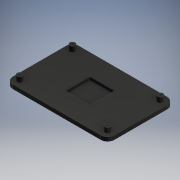
# Autodesk Inventor part: BackBracket
Saved by Autodesk Inventor 2018 (Build 220112000, 112)
## iProperties
Created: 2020-01-28
Part Number: BackBracket
Material: Steel, Mild
Document SubType Name: Modeling
Designer: Bradley
Density: 7.85 g/cm^3
Appearance: Glossy - Black
Author: Bradley
Autodesk Inventor part; units mm, degrees
ref_plane "YZ Plane" through (0, 0, 0) normal (1, 0, 0) x (0, 1, 0)
ref_plane "XZ Plane" through (0, 0, 0) normal (0, 1, 0) x (-1, 0, 0)
ref_plane "XY Plane" through (0, 0, 0) normal (0, 0, 1) x (1, 0, 0)
sketch "Sketch1" plane through (0, 0, 0) normal (0, 0, 1) x (1, 0, 0)
  line L0 (-45, -34) -> (45, -34)
  line L1 (52, -27) -> (52, 27)
  line L2 (45, 34) -> (-45, 34)
  line L3 (-52, 27) -> (-52, -27)
  line L4 (-52, -34) -> (52, 34) construction
  line L5 (52, -34) -> (-52, 34) construction
  line L6 (-45, 27) -> (45, 27) construction
  line L7 (45, 27) -> (45, -27) construction
  line L8 (45, -27) -> (-45, -27) construction
  line L9 (-45, -27) -> (-45, 27) construction
  arc A0 (-45, 34) -> (-52, 27) centre (-45, 27) ccw
  arc A1 (52, 27) -> (45, 34) centre (45, 27) ccw
  arc A2 (45, -34) -> (52, -27) centre (45, -27) ccw
  arc A3 (-52, -27) -> (-45, -34) centre (-45, -27) ccw
  point P0 (0, 0)
  dimension "d0" = 104
  dimension "d1" = 68
  dimension "d2" = 54
  dimension "d3" = 90
  constraints: 20 end point, 8 point on circle, 8 point on line, 8 tangent, 4 centre point, 4 parallel, 3 equal radius, 2 midpoint, 2 perpendicular, 1 coincident, 1 horizontal, 3 other
  measures "d0" distance of L5.end L4.end
  measures "d1" distance of L4.end L5.start
  measures "d2" distance of L8.end L6.start
  measures "d3" distance of L6.start L6.end
extrude "Extrusion1" add sketch "Sketch1" along normal mid plane 4
sketch "Sketch2" plane through (0, 0, 2) normal (0, 0, 1) x (1, 0, 0)
  line L0 (45, 34) -> (-45, 34) projected
  arc A0 (-45, 34) -> (-52, 27) centre (-45, 27) ccw projected
  line L1 (-52, 27) -> (-52, -27) projected
  arc A1 (-52, -27) -> (-45, -34) centre (-45, -27) ccw projected
  line L2 (-45, -34) -> (45, -34) projected
  arc A2 (45, -34) -> (52, -27) centre (45, -27) ccw projected
  line L3 (52, -27) -> (52, 27) projected
  arc A3 (52, 27) -> (45, 34) centre (45, 27) ccw projected
  circle A4 centre (-45, 27) radius 2.75
  circle A5 centre (45, 27) radius 2.75
  circle A6 centre (45, -27) radius 2.75
  circle A7 centre (-45, -27) radius 2.75
  point P0 (0, 0)
  dimension "d7" = 5.5
  constraints: 4 centre point, 4 coincident, 3 equal radius
  measures "d7" diameter of A4
extrude "Extrusion2" add sketch "Sketch2" along normal blind 5.3 contours A4 | A5 | A6 | A7
sketch "Sketch3" plane through (0, 0, -2) normal (0, 0, -1) x (-1, 0, 0)
  line L0 (45, 34) -> (-45, 34) projected
  arc A0 (-45, 34) -> (-52, 27) centre (-45, 27) ccw projected
  line L1 (-52, 27) -> (-52, -27) projected
  arc A1 (-52, -27) -> (-45, -34) centre (-45, -27) ccw projected
  line L2 (-45, -34) -> (45, -34) projected
  arc A2 (45, -34) -> (52, -27) centre (45, -27) ccw projected
  line L3 (52, -27) -> (52, 27) projected
  arc A3 (52, 27) -> (45, 34) centre (45, 27) ccw projected
  circle A4 centre (-45, 27) radius 2.75 projected
  point P0 (0, 0)
  constraints: 4 coincident
hole "Hole1" at (-45, -27, -2) at (45, -27, -2) at (45, 27, -2) at (-45, 27, -2) direction (0, 0, 1) diameter 2.642 end through all thread size "6-32 UNC" class "2B" standard "ANSI Unified Screw Threads"
sketch "Sketch4" plane through (0, 0, 2) normal (0, 0, 1) x (1, 0, 0)
  line L0 (-12.5, -12.5) -> (12.5, -12.5)
  line L1 (12.5, -12.5) -> (12.5, 12.5)
  line L2 (12.5, 12.5) -> (-12.5, 12.5)
  line L3 (-12.5, 12.5) -> (-12.5, -12.5)
  line L4 (-12.5, -12.5) -> (12.5, 12.5) construction
  line L5 (12.5, -12.5) -> (-12.5, 12.5) construction
  point P0 (0, 0)
  dimension "d17" = 25
  constraints: 12 end point, 2 midpoint, 2 parallel, 2 perpendicular, 1 horizontal
  measures "d17" distance of L2.end L1.end
extrude "Extrusion3" cut sketch "Sketch4" against normal blind 3.35
body "Solid1"
